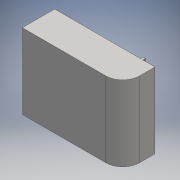
# Autodesk Inventor part: boxgeneric
Saved by Autodesk Inventor 2016 (Build 200138000, 138)
## iProperties
Created: 2015-12-29
Part Number: boxgeneric
Material: Generic
Document SubType Name: Modeling
Designer: hesaon
Density: 1 g/cm^3
Appearance: Default
Author: hesaon
Autodesk Inventor part; units mm, degrees
ref_plane "YZ Plane" through (0, 0, 0) normal (1, 0, 0) x (0, 1, 0)
ref_plane "XZ Plane" through (0, 0, 0) normal (0, 1, 0) x (-1, 0, 0)
ref_plane "XY Plane" through (0, 0, 0) normal (0, 0, 1) x (1, 0, 0)
sketch "Sketch1" plane through (0, 0, 0) normal (0, 0, 1) x (1, 0, 0)
  line L0 (0, 0) -> (110, 0)
  line L1 (0, 42.5) -> (0, 0)
  line L2 (132, 42.5) -> (116, 42.5)
  line L3 (116, 42.5) -> (116, 46)
  line L4 (116, 46) -> (113, 46)
  line L5 (113, 46) -> (113, 42.5)
  line L6 (113, 42.5) -> (110, 42.5)
  arc A0 (110, 0) -> (132, 22) centre (110, 22) ccw
  line L7 (110, 22) -> (110, 0) construction
  line L8 (132, 22) -> (132, 42.5)
  line L9 (132, 42.5) -> (116, 42.5)
  line L10 (113, 42.5) -> (0, 42.5)
  dimension "d2" = 16
  dimension "d3" = 3.5
  dimension "thickness" = 3
  dimension "d5" = 3
  dimension "d14" = 110
  dimension "d15" = 22
  dimension "d16" = 22
  dimension "height" = 20.5
  dimension "d18" = 110
  dimension "d19" = 90
  dimension "d20" = 3
  constraints: 22 end point, 6 perpendicular, 2 point on circle, 1 centre point, 1 horizontal, 1 point on line, 1 vertical
  measures "d2" distance of L2.start L2.end
  measures "d3" distance of L2.end L3.end
  measures "thickness" distance of L3.end L4.end
  measures "d5" distance of L5.end L6.end
  measures "d14" distance of L0.start L0.end
  measures "d15" distance of L7.start L8.start
  measures "d16" horizontal distance of L8.start L0.end
  measures "height" distance of L8.start L2.start
  measures "d18" distance of L6.end L1.start
  measures "d20" distance of L2.end L5.end
extrude "Extrusion1" add sketch "Sketch1" along normal blind 3
sketch "Sketch2" plane through (0, 0, 3) normal (0, 0, 1) x (1, 0, 0)
  line L0 (0, 42.5) -> (3, 42.5)
  line L1 (113, 42.5) -> (0, 42.5) projected
  line L2 (3, 42.5) -> (3, 15)
  line L3 (0, 0) -> (110, 0) projected
  line L4 (4, 42.5) -> (4, 15)
  line L5 (4, 42.5) -> (7, 42.5)
  line L6 (7, 42.5) -> (7, 3)
  line L7 (0, 42.5) -> (0, 0) projected
  line L8 (0, 0) -> (0, 15)
  line L9 (3, 15) -> (4, 15)
  line L10 (0, 42.5) -> (0, 15)
  line L11 (132, 42.5) -> (129, 42.5)
  line L12 (132, 42.5) -> (116, 42.5) projected
  line L13 (129, 42.5) -> (129, 22)
  arc A0 (110, 0) -> (132, 22) centre (110, 22) ccw projected
  line L14 (132, 22) -> (132, 42.5) projected
  line L15 (132, 22) -> (132, 42.5)
  line L16 (7, 0) -> (110, 0)
  line L17 (7, 3) -> (110, 3)
  line L18 (129, 22) -> (129, 22)
  arc A1 (110, 3) -> (129, 22) centre (110, 22) ccw
  arc A2 (110, 0) -> (132, 22) centre (110, 22) ccw
  line L19 (0, 0) -> (7, 0)
  dimension "d27" = 27.5
  dimension "d28" = 3
  dimension "d29" = 3
  dimension "d35" = 3
  dimension "d36" = 3
  dimension "d37" = 3
  dimension "d38" = 20.5
  dimension "d39" = 103
  dimension "d40" = 103
  dimension "d41" = 1
  dimension "d42" = 27.5
  dimension "d43" = 1
  constraints: 30 end point, 7 point on line, 4 point on circle, 3 collinear, 3 perpendicular, 2 centre point, 2 coincident, 2 tangent, 1 parallel, 1 vertical
  measures "d27" distance of L8.end L0.start
  measures "d28" distance of L0.end L0.start
  measures "d29" distance of L5.end L4.start
  measures "d35" distance of L14.start L13.end
  measures "d36" distance of L11.start L11.end
  measures "d37" distance of L3.end L17.end
  measures "d38" distance of L11.start L14.start
  measures "d39" distance of L3.end L16.start
  measures "d40" distance of L6.end L17.end
  measures "d41" distance of L4.start L0.end
  measures "d42" distance of L4.start L4.end
  measures "d43" distance of L4.end L2.end
extrude "Extrusion2" add sketch "Sketch2" along normal blind 3 contours L0 L2 L9 L4 L1 L6 L17 A1 L13 L11 L14 A0 L3 L7
sketch "Sketch3" plane through (0, 0, 6) normal (0, 0, 1) x (1, 0, 0)
  line L0 (113, 42.5) -> (7, 42.5) projected
  line L1 (4, 42.5) -> (4, 15) projected
  line L2 (7, 42.5) -> (4, 42.5)
  line L3 (4, 42.5) -> (4, 15)
  line L4 (3, 42.5) -> (3, 15) projected
  line L5 (4, 15) -> (3, 15)
  line L6 (3, 15) -> (0, 15)
  line L7 (0, 42.5) -> (0, 0) projected
  line L8 (0, 15) -> (0, 0)
  line L9 (0, 0) -> (7, 0)
  line L10 (0, 0) -> (110, 0) projected
  arc A0 (110, 0) -> (132, 22) centre (110, 22) ccw projected
  line L11 (132, 22) -> (132, 42.5) projected
  line L12 (132, 22) -> (132, 42.5)
  line L13 (132, 42.5) -> (128.8778, 42.5)
  line L14 (132, 42.5) -> (116, 42.5) projected
  line L15 (7, 42.5) -> (7, 3) projected
  line L16 (7, 42.5) -> (7, 3)
  line L17 (110, 3) -> (7, 3) projected
  line L18 (7, 3) -> (110, 3)
  line L19 (129, 42.5) -> (129, 22) projected
  line L20 (129, 42.5) -> (129, 22)
  arc A1 (110, 3) -> (129, 22) centre (110, 22) ccw
  arc A2 (110, 0) -> (132, 22) centre (110, 22) ccw
  line L21 (7, 0) -> (110, 0)
  constraints: 24 end point, 4 collinear, 4 point on circle, 3 point on line, 2 centre point, 2 coincident, 2 horizontal, 2 perpendicular, 1 parallel, 1 tangent
extrude "Extrusion3" add sketch "Sketch3" along normal blind 87
sketch "Sketch5" plane through (0, 0, 93) normal (0, 0, 1) x (1, 0, 0)
  arc A0 (110, 3) -> (129, 22) centre (110, 22) ccw projected
  arc A1 (110, 3) -> (129, 22) centre (110, 22) ccw
  arc A2 (110, 0) -> (132, 22) centre (110, 22) ccw
  line L0 (132, 22) -> (132, 42.5) projected
  line L1 (132, 22) -> (132, 42.5)
  line L2 (132, 42.5) -> (129, 42.5)
  line L3 (129, 22) -> (129, 42.5) projected
  line L4 (129, 42.5) -> (129, 22)
  line L5 (7, 42.5) -> (7, 3) projected
  line L6 (110, 3) -> (7, 3)
  line L7 (7, 3) -> (7, 42.5)
  line L8 (7, 42.5) -> (4, 42.5)
  line L9 (4, 15) -> (0, 15) projected
  line L10 (4, 42.5) -> (4, 15)
  line L11 (3, 15) -> (3, 42.5) projected
  line L12 (4, 15) -> (3, 15)
  line L13 (3, 15) -> (3, 42.5)
  line L14 (113, 42.5) -> (0, 42.5) projected
  line L15 (3, 42.5) -> (0, 42.5)
  line L16 (0, 15) -> (0, 0) projected
  line L17 (0, 42.5) -> (0, 15)
  line L18 (0, 0) -> (110, 0) projected
  line L19 (0, 15) -> (0, 0)
  line L20 (0, 0) -> (110, 0)
  line L21 (3, 42.5) -> (0, 42.5)
  line L22 (0, 42.5) -> (0, 15)
  line L23 (3, 15) -> (3, 42.5)
  line L24 (3, 15) -> (0, 15)
  dimension "d52" = 3
  constraints: 34 end point, 9 perpendicular, 4 collinear, 4 point on circle, 2 centre point, 2 coincident, 2 horizontal, 1 parallel, 1 vertical
  measures "d52" distance from line of A1.end L0
extrude "Extrusion4" add sketch "Sketch5" along normal blind 3 contours A0 L3 L2 L0 A2 L18 L16 L9 L10 L8 L5 L6 | L11 L9 L17 L14
sketch "Sketch6" plane through (0, 0, 96) normal (0, 0, 1) x (1, 0, 0)
  line L0 (132, 22) -> (132, 42.5) projected
  line L1 (129, 22) -> (129, 42.5) projected
  line L2 (132, 42.5) -> (129, 42.5)
  line L3 (132, 22) -> (132, 42.5)
  line L4 (7, 42.5) -> (7, 3) projected
  line L5 (0, 42.5) -> (0, 0) projected
  line L6 (7, 42.5) -> (0, 42.5)
  line L7 (0, 42.5) -> (0, 0)
  line L8 (0, 0) -> (7, 0)
  arc A0 (110, 0) -> (132, 22) centre (110, 22) ccw projected
  line L9 (110, 0) -> (7, 0)
  line L10 (0, 0) -> (110, 0) projected
  arc A1 (110, 0) -> (132, 22) centre (110, 22) ccw
  line L11 (7, 42.5) -> (4, 42.5) projected
  line L12 (132, 42.5) -> (116, 42.5) projected
  line L13 (116, 42.5) -> (116, 46) projected
  line L14 (116, 42.5) -> (116, 46)
  line L15 (116, 46) -> (113, 46) projected
  line L16 (116, 46) -> (113, 46)
  line L17 (113, 46) -> (113, 42.5) projected
  line L18 (113, 46) -> (113, 42.5)
  line L19 (129, 42.5) -> (116, 42.5)
  line L20 (113, 42.5) -> (7, 42.5)
  dimension "d55" = 125
  dimension "d56" = 125
  dimension "d57" = 22
  dimension "d58" = 90
  dimension "d59" = 90
  dimension "d60" = 20.5
  dimension "d61" = 3
  constraints: 22 end point, 4 equal length, 4 horizontal, 2 point on circle, 1 centre point, 1 perpendicular
  measures "d55" distance from line of L9.end L0
  measures "d56" distance from line of L8.end L0
  measures "d57" radius of A1
  measures "d58" angle of L12 L3
  measures "d59" angle of L0 L9
  measures "d60" distance from line of L3.start L12
  measures "d61" distance from line of L2.end L0
extrude "Extrusion5" add sketch "Sketch6" along normal blind 3
equation "\"d5\" = thickness"
equation "\"d20\" = thickness"
equation "\"d21\" = thickness"
equation "\"d28\" = thickness"
equation "\"d29\" = thickness"
equation "\"d35\" = thickness"
equation "\"d36\" = thickness"
equation "\"d37\" = thickness"
equation "\"d38\" = height"
equation "\"d44\" = thickness"
equation "\"d53\" = thickness"
equation "\"d62\" = thickness"
body "Solid1"
